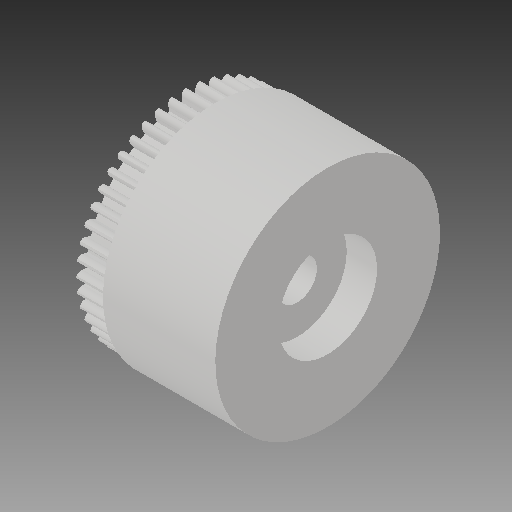
# Autodesk Inventor part: correct_wheel
Saved by Autodesk Inventor 2018 (Build 220112000, 112)
## iProperties
Created: 2017-11-06
Part Number: correct_wheel
Material: Generic
Document SubType Name: Modeling
Designer: kcmat
Density: 1 g/cm^3
Appearance: Default
Author: kcmat
Autodesk Inventor part; units mm, degrees
ref_plane "YZ Plane" through (0, 0, 0) normal (1, 0, 0) x (0, 1, 0)
ref_plane "XZ Plane" through (0, 0, 0) normal (0, 1, 0) x (-1, 0, 0)
ref_plane "XY Plane" through (0, 0, 0) normal (0, 0, 1) x (1, 0, 0)
sketch "Sketch1" plane through (0, 0, 0) normal (1, 0, 0) x (0, 1, 0)
  circle A0 centre (0, 0) radius 25.4
  circle A1 centre (0, 0) radius 4.445
  dimension "d3" = 8.89
  constraints: 2 centre point, 1 coincident
  measures "d3" diameter of A1
extrude "Extrusion1" add sketch "Sketch1" along normal blind 25.4
sketch "Sketch2" plane through (0, 0, 0) normal (-1, 0, 0) x (0, 0, 1)
  circle A0 centre (0, 0) radius 10.9855
  dimension "d6" = 21.971
  constraints: 1 centre point, 1 coincident
  measures "d6" diameter of A0
extrude "Extrusion2" cut sketch "Sketch2" against normal blind 6.858
sketch "Sketch3" plane through (25.4, 0, 0) normal (1, 0, 0) x (0, 0, -1)
  circle A0 centre (0, 0) radius 10.9855
  dimension "d9" = 21.971
  constraints: 1 centre point, 1 coincident
  measures "d9" diameter of A0
extrude "Extrusion3" cut sketch "Sketch3" against normal blind 6.858
sketch "Sketch4" plane through (0, 0, 0) normal (-1, 0, 0) x (0, 0, 1)
  circle A0 centre (0, 0) radius 10.9855
  circle A1 centre (0, 0) radius 10.9855 projected
  line L0 (-22.3513, -1.1327) -> (-22.3431, -1.1327) construction
  arc A2 (-24.7744, 0.2429) -> (-24.7744, -0.246) centre (-0.1732, -0.0016) ccw
  line L1 (-22.38, 1.002) -> (-22.3575, 0.9992)
  circle A3 centre (-0.1732, -0.0016) radius 22.2128
  arc A4 (-22.38, 0.5127) -> (-22.38, -0.5158) centre (-0.1732, -0.0016) ccw
  arc A5 (-24.7744, -0.246) -> (-23.3358, -0.7286) centre (-23.7217, 0.5066) ccw
  line L2 (-23.3358, -0.7286) -> (-22.3763, -0.6565)
  arc A6 (-23.3358, 0.7254) -> (-24.7744, 0.2429) centre (-23.7217, -0.5097) ccw
  line L3 (-23.3358, 0.7254) -> (-22.3763, 0.6534)
  arc A7 (-22.3763, 0.6534) -> (-22.3763, -0.6565) centre (-0.1732, -0.0016) ccw
  line L4 (-22.0139, -4.0179) -> (-22.0057, -4.0168) construction
  arc A8 (-22.2571, -2.3903) -> (-22.1229, -3.41) centre (-0.1732, -0.0016) ccw
  arc A9 (-22.2718, -2.2503) -> (-22.1009, -3.549) centre (-0.1732, -0.0016) ccw
  line L5 (-23.0427, -3.7457) -> (-22.1009, -3.549)
  line L6 (-23.2325, -2.3041) -> (-22.2718, -2.2503)
  arc A10 (-24.5321, -3.4551) -> (-23.0427, -3.7457) centre (-23.5866, -2.5715) ccw
  arc A11 (-24.5959, -2.9703) -> (-24.5321, -3.4551) centre (-0.1732, -0.0016) ccw
  arc A12 (-23.2325, -2.3041) -> (-24.5959, -2.9703) centre (-23.454, -3.5791) ccw
  line L7 (-22.321, -1.9052) -> (-22.2984, -1.905)
  line L8 (-21.3028, -6.8343) -> (-21.2949, -6.8322) construction
  arc A13 (-21.7564, -5.2524) -> (-21.4902, -6.2458) centre (-0.1732, -0.0016) ccw
  arc A14 (-21.7892, -5.1156) -> (-21.4502, -6.3807) centre (-0.1732, -0.0016) ccw
  line L9 (-22.3583, -6.6987) -> (-21.4502, -6.3807)
  line L10 (-22.7347, -5.2942) -> (-21.7892, -5.1156)
  arc A15 (-23.8729, -6.605) -> (-22.3583, -6.6987) centre (-23.0509, -5.6055) ccw
  arc A16 (-23.9994, -6.1327) -> (-23.8729, -6.605) centre (-0.1732, -0.0016) ccw
  arc A17 (-22.7347, -5.2942) -> (-23.9994, -6.1327) centre (-22.7878, -6.5872) ccw
  line L11 (-21.8831, -4.7797) -> (-21.8607, -4.7766)
  line L12 (-20.2302, -9.5338) -> (-20.2226, -9.5307) construction
  arc A18 (-20.8864, -8.0247) -> (-20.4928, -8.9748) centre (-0.1732, -0.0016) ccw
  arc A19 (-20.9368, -7.8933) -> (-20.4356, -9.1034) centre (-0.1732, -0.0016) ccw
  line L13 (-21.2944, -9.5372) -> (-20.4356, -9.1034)
  line L14 (-21.8508, -8.1938) -> (-20.9368, -7.8933)
  arc A20 (-22.8082, -9.6419) -> (-21.2944, -9.5372) centre (-22.1237, -8.5437) ccw
  arc A21 (-22.9953, -9.1902) -> (-22.8082, -9.6419) centre (-0.1732, -0.0016) ccw
  arc A22 (-21.8508, -8.1938) -> (-22.9953, -9.1902) centre (-21.7348, -9.4827) ccw
  line L15 (-21.0737, -7.5726) -> (-21.0518, -7.5665)
  line L16 (-18.8144, -12.0703) -> (-18.8073, -12.0661) construction
  arc A23 (-19.662, -10.6596) -> (-19.1477, -11.5503) centre (-0.1732, -0.0016) ccw
  arc A24 (-19.7291, -10.5359) -> (-19.0742, -11.6703) centre (-0.1732, -0.0016) ccw
  line L17 (-19.8691, -12.2125) -> (-19.0742, -11.6703)
  line L18 (-20.5961, -10.9532) -> (-19.7291, -10.5359)
  arc A25 (-21.3562, -12.5139) -> (-19.8691, -12.2125) centre (-20.8209, -11.3358) ccw
  arc A26 (-21.6007, -12.0905) -> (-21.3562, -12.5139) centre (-0.1732, -0.0016) ccw
  arc A27 (-20.5961, -10.9532) -> (-21.6007, -12.0905) centre (-20.3128, -12.2159) ccw
  line L19 (-19.9066, -10.2359) -> (-19.8858, -10.227)
  line L20 (-17.0796, -14.4002) -> (-17.0731, -14.3952) construction
  arc A28 (-18.1041, -13.1123) -> (-17.478, -13.9282) centre (-0.1732, -0.0016) ccw
  arc A29 (-18.1868, -12.9984) -> (-17.3894, -14.0375) centre (-0.1732, -0.0016) ccw
  line L21 (-18.1067, -14.6788) -> (-17.3894, -14.0375)
  line L22 (-18.9919, -13.5253) -> (-18.1868, -12.9984)
  arc A30 (-19.5418, -15.1718) -> (-18.1067, -14.6788) centre (-19.1649, -13.9339) ccw
  arc A31 (-19.8395, -14.7839) -> (-19.5418, -15.1718) centre (-0.1732, -0.0016) ccw
  arc A32 (-18.9919, -13.5253) -> (-19.8395, -14.7839) centre (-18.5462, -14.7402) ccw
  line L23 (-18.402, -12.724) -> (-18.3825, -12.7126)
  line L24 (-15.0556, -16.4837) -> (-15.0498, -16.4779) construction
  arc A33 (-16.2394, -15.3405) -> (-15.5122, -16.0678) centre (-0.1732, -0.0016) ccw
  arc A34 (-16.3362, -15.2384) -> (-15.4101, -16.1646) centre (-0.1732, -0.0016) ccw
  line L25 (-16.0375, -16.894) -> (-15.4101, -16.1646)
  line L26 (-17.0657, -15.8659) -> (-16.3362, -15.2384)
  arc A35 (-17.396, -17.5701) -> (-16.0375, -16.894) centre (-17.1838, -16.2936) ccw
  arc A36 (-17.7418, -17.2244) -> (-17.396, -17.5701) centre (-0.1732, -0.0016) ccw
  arc A37 (-17.0657, -15.8659) -> (-17.7418, -17.2244) centre (-16.4652, -17.0122) ccw
  line L27 (-16.5854, -14.9945) -> (-16.5676, -14.9806)
  line L28 (-12.7769, -18.2853) -> (-12.7719, -18.2787) construction
  arc A38 (-14.0998, -17.3064) -> (-13.2839, -17.9325) centre (-0.1732, -0.0016) ccw
  arc A39 (-14.2092, -17.2178) -> (-13.17, -18.0152) centre (-0.1732, -0.0016) ccw
  line L29 (-13.6969, -18.8202) -> (-13.17, -18.0152)
  line L30 (-14.8504, -17.9351) -> (-14.2092, -17.2178)
  arc A40 (-14.9555, -19.6679) -> (-13.6969, -18.8202) centre (-14.9118, -18.3745) ccw
  arc A41 (-15.3434, -19.3702) -> (-14.9555, -19.6679) centre (-0.1732, -0.0016) ccw
  arc A42 (-14.8504, -17.9351) -> (-15.3434, -19.3702) centre (-14.1055, -18.9932) ccw
  line L31 (-14.488, -17.0085) -> (-14.4722, -16.9923)
  line L32 (-10.2826, -19.774) -> (-10.2785, -19.7668) construction
  arc A43 (-11.7219, -18.9761) -> (-10.8313, -19.4903) centre (-0.1732, -0.0016) ccw
  arc A44 (-11.8419, -18.9026) -> (-10.7076, -19.5575) centre (-0.1732, -0.0016) ccw
  line L33 (-11.1249, -20.4244) -> (-10.7076, -19.5575)
  line L34 (-12.3841, -19.6974) -> (-11.8419, -18.9026)
  arc A45 (-12.2621, -21.4291) -> (-11.1249, -20.4244) centre (-12.3875, -20.1411) ccw
  arc A46 (-12.6855, -21.1846) -> (-12.2621, -21.4291) centre (-0.1732, -0.0016) ccw
  arc A47 (-12.3841, -19.6974) -> (-12.6855, -21.1846) centre (-11.5074, -20.6493) ccw
  line L35 (-12.1457, -18.7315) -> (-12.1321, -18.7134)
  line L36 (-7.6153, -20.9244) -> (-7.6121, -20.9167) construction
  arc A48 (-9.1464, -20.3212) -> (-8.1963, -20.7148) centre (-0.1732, -0.0016) ccw
  arc A49 (-9.275, -20.2639) -> (-8.0649, -20.7652) centre (-0.1732, -0.0016) ccw
  line L37 (-8.3654, -21.6792) -> (-8.0649, -20.7652)
  line L38 (-9.7088, -21.1228) -> (-9.275, -20.2639)
  arc A50 (-9.3618, -22.8237) -> (-8.3654, -21.6792) centre (-9.6543, -21.5631) ccw
  arc A51 (-9.8135, -22.6366) -> (-9.3618, -22.8237) centre (-0.1732, -0.0016) ccw
  arc A52 (-9.7088, -21.1228) -> (-9.8135, -22.6366) centre (-8.7153, -21.9521) ccw
  line L39 (-9.5985, -20.1339) -> (-9.5874, -20.1142)
  line L40 (-4.8207, -21.7168) -> (-4.8185, -21.7088) construction
  arc A53 (-6.4174, -21.3186) -> (-5.424, -21.5848) centre (-0.1732, -0.0016) ccw
  arc A54 (-6.5524, -21.2786) -> (-5.2872, -21.6176) centre (-0.1732, -0.0016) ccw
  line L41 (-5.4659, -22.5631) -> (-5.2872, -21.6176)
  line L42 (-6.8703, -22.1867) -> (-6.5524, -21.2786)
  arc A55 (-6.3043, -23.8278) -> (-5.4659, -22.5631) centre (-6.7588, -22.6162) ccw
  arc A56 (-6.7766, -23.7013) -> (-6.3043, -23.8278) centre (-0.1732, -0.0016) ccw
  arc A57 (-6.8703, -22.1867) -> (-6.7766, -23.7013) centre (-5.7772, -22.8792) ccw
  line L43 (-6.8901, -21.192) -> (-6.8816, -21.171)
  line L44 (-1.9465, -22.1376) -> (-1.9454, -22.1294) construction
  arc A58 (-3.5816, -21.9513) -> (-2.5619, -22.0855) centre (-0.1732, -0.0016) ccw
  arc A59 (-3.7206, -21.9292) -> (-2.422, -22.1002) centre (-0.1732, -0.0016) ccw
  line L45 (-2.4757, -23.0609) -> (-2.422, -22.1002)
  line L46 (-3.9173, -22.8711) -> (-3.7206, -21.9292)
  arc A60 (-3.1419, -24.4243) -> (-2.4757, -23.0609) centre (-3.7507, -23.2823) ccw
  arc A61 (-3.6267, -24.3604) -> (-3.1419, -24.4243) centre (-0.1732, -0.0016) ccw
  arc A62 (-3.9173, -22.8711) -> (-3.6267, -24.3604) centre (-2.7431, -23.415) ccw
  line L47 (-4.0667, -21.8874) -> (-4.0611, -21.8655)
  line L48 (0.958, -22.1797) -> (0.958, -22.1714) construction
  arc A63 (-0.6874, -22.2084) -> (0.341, -22.2084) centre (-0.1732, -0.0016) ccw
  arc A64 (-0.8281, -22.2047) -> (0.4817, -22.2047) centre (-0.1732, -0.0016) ccw
  line L49 (0.5538, -23.1641) -> (0.4817, -22.2047)
  line L50 (-0.9002, -23.1641) -> (-0.8281, -22.2047)
  arc A65 (0.0713, -24.6028) -> (0.5538, -23.1641) centre (-0.6813, -23.5501) ccw
  arc A66 (-0.4177, -24.6028) -> (0.0713, -24.6028) centre (-0.1732, -0.0016) ccw
  arc A67 (-0.9002, -23.1641) -> (-0.4177, -24.6028) centre (0.335, -23.5501) ccw
  line L51 (-1.1767, -22.2084) -> (-1.174, -22.1859)
  line L52 (3.8432, -21.8423) -> (3.8421, -21.8341) construction
  arc A68 (2.2156, -22.0855) -> (3.2352, -21.9513) centre (-0.1732, -0.0016) ccw
  arc A69 (2.0756, -22.1002) -> (3.3742, -21.9292) centre (-0.1732, -0.0016) ccw
  line L53 (3.5709, -22.8711) -> (3.3742, -21.9292)
  line L54 (2.1294, -23.0609) -> (2.0756, -22.1002)
  arc A70 (3.2803, -24.3604) -> (3.5709, -22.8711) centre (2.3967, -23.415) ccw
  arc A71 (2.7955, -24.4243) -> (3.2803, -24.3604) centre (-0.1732, -0.0016) ccw
  arc A72 (2.1294, -23.0609) -> (2.7955, -24.4243) centre (3.4043, -23.2823) ccw
  line L55 (1.7304, -22.1494) -> (1.7302, -22.1268)
  line L56 (6.6596, -21.1312) -> (6.6575, -21.1232) construction
  arc A73 (5.0777, -21.5848) -> (6.0711, -21.3186) centre (-0.1732, -0.0016) ccw
  arc A74 (4.9408, -21.6176) -> (6.206, -21.2786) centre (-0.1732, -0.0016) ccw
  line L57 (6.524, -22.1867) -> (6.206, -21.2786)
  line L58 (5.1195, -22.5631) -> (4.9408, -21.6176)
  arc A75 (6.4302, -23.7013) -> (6.524, -22.1867) centre (5.4308, -22.8792) ccw
  arc A76 (5.9579, -23.8278) -> (6.4302, -23.7013) centre (-0.1732, -0.0016) ccw
  arc A77 (5.1195, -22.5631) -> (5.9579, -23.8278) centre (6.4125, -22.6162) ccw
  line L59 (4.605, -21.7114) -> (4.6019, -21.689)
  line L60 (9.3591, -20.0586) -> (9.356, -20.051) construction
  arc A78 (7.8499, -20.7148) -> (8.8001, -20.3212) centre (-0.1732, -0.0016) ccw
  arc A79 (7.7185, -20.7652) -> (8.9286, -20.2639) centre (-0.1732, -0.0016) ccw
  line L61 (9.3624, -21.1228) -> (8.9286, -20.2639)
  line L62 (8.0191, -21.6792) -> (7.7185, -20.7652)
  arc A80 (9.4672, -22.6366) -> (9.3624, -21.1228) centre (8.369, -21.9521) ccw
  arc A81 (9.0154, -22.8237) -> (9.4672, -22.6366) centre (-0.1732, -0.0016) ccw
  arc A82 (8.0191, -21.6792) -> (9.0154, -22.8237) centre (9.3079, -21.5631) ccw
  line L63 (7.3978, -20.902) -> (7.3918, -20.8802)
  line L64 (11.8955, -18.6428) -> (11.8914, -18.6356) construction
  arc A83 (10.4849, -19.4903) -> (11.3756, -18.9761) centre (-0.1732, -0.0016) ccw
  arc A84 (10.3612, -19.5575) -> (11.4956, -18.9026) centre (-0.1732, -0.0016) ccw
  line L65 (12.0377, -19.6974) -> (11.4956, -18.9026)
  line L66 (10.7785, -20.4244) -> (10.3612, -19.5575)
  arc A85 (12.3392, -21.1846) -> (12.0377, -19.6974) centre (11.161, -20.6493) ccw
  arc A86 (11.9157, -21.4291) -> (12.3392, -21.1846) centre (-0.1732, -0.0016) ccw
  arc A87 (10.7785, -20.4244) -> (11.9157, -21.4291) centre (12.0412, -20.1411) ccw
  line L67 (10.0611, -19.735) -> (10.0523, -19.7142)
  line L68 (14.2254, -16.908) -> (14.2204, -16.9015) construction
  arc A88 (12.9375, -17.9325) -> (13.7534, -17.3064) centre (-0.1732, -0.0016) ccw
  arc A89 (12.8236, -18.0152) -> (13.8628, -17.2178) centre (-0.1732, -0.0016) ccw
  line L69 (14.5041, -17.9351) -> (13.8628, -17.2178)
  line L70 (13.3505, -18.8202) -> (12.8236, -18.0152)
  arc A90 (14.9971, -19.3702) -> (14.5041, -17.9351) centre (13.7591, -18.9932) ccw
  arc A91 (14.6092, -19.6679) -> (14.9971, -19.3702) centre (-0.1732, -0.0016) ccw
  arc A92 (13.3505, -18.8202) -> (14.6092, -19.6679) centre (14.5654, -18.3745) ccw
  line L71 (12.5493, -18.2303) -> (12.5378, -18.2108)
  line L72 (16.309, -14.884) -> (16.3032, -14.8782) construction
  arc A93 (15.1658, -16.0678) -> (15.893, -15.3405) centre (-0.1732, -0.0016) ccw
  arc A94 (15.0637, -16.1646) -> (15.9899, -15.2384) centre (-0.1732, -0.0016) ccw
  line L73 (16.7193, -15.8659) -> (15.9899, -15.2384)
  line L74 (15.6912, -16.894) -> (15.0637, -16.1646)
  arc A95 (17.3954, -17.2244) -> (16.7193, -15.8659) centre (16.1189, -17.0122) ccw
  arc A96 (17.0497, -17.5701) -> (17.3954, -17.2244) centre (-0.1732, -0.0016) ccw
  arc A97 (15.6912, -16.894) -> (17.0497, -17.5701) centre (16.8375, -16.2936) ccw
  line L75 (14.8198, -16.4138) -> (14.8059, -16.3959)
  line L76 (18.1105, -12.6053) -> (18.104, -12.6003) construction
  arc A98 (17.1316, -13.9282) -> (17.7577, -13.1123) centre (-0.1732, -0.0016) ccw
  arc A99 (17.0431, -14.0375) -> (17.8404, -12.9984) centre (-0.1732, -0.0016) ccw
  line L77 (18.6455, -13.5253) -> (17.8404, -12.9984)
  line L78 (17.7604, -14.6788) -> (17.0431, -14.0375)
  arc A100 (19.4931, -14.7839) -> (18.6455, -13.5253) centre (18.1998, -14.7402) ccw
  arc A101 (19.1955, -15.1718) -> (19.4931, -14.7839) centre (-0.1732, -0.0016) ccw
  arc A102 (17.7604, -14.6788) -> (19.1955, -15.1718) centre (18.8185, -13.9339) ccw
  line L79 (16.8338, -14.3164) -> (16.8176, -14.3005)
  line L80 (19.5992, -10.111) -> (19.5921, -10.1069) construction
  arc A103 (18.8014, -11.5503) -> (19.3156, -10.6596) centre (-0.1732, -0.0016) ccw
  arc A104 (18.7278, -11.6703) -> (19.3827, -10.5359) centre (-0.1732, -0.0016) ccw
  line L81 (20.2497, -10.9532) -> (19.3827, -10.5359)
  line L82 (19.5227, -12.2125) -> (18.7278, -11.6703)
  arc A105 (21.2544, -12.0905) -> (20.2497, -10.9532) centre (19.9664, -12.2159) ccw
  arc A106 (21.0099, -12.5139) -> (21.2544, -12.0905) centre (-0.1732, -0.0016) ccw
  arc A107 (19.5227, -12.2125) -> (21.0099, -12.5139) centre (20.4746, -11.3358) ccw
  line L83 (18.5567, -11.9741) -> (18.5386, -11.9605)
  line L84 (20.7496, -7.4437) -> (20.742, -7.4405) construction
  arc A108 (20.1465, -8.9748) -> (20.54, -8.0247) centre (-0.1732, -0.0016) ccw
  arc A109 (20.0892, -9.1034) -> (20.5905, -7.8933) centre (-0.1732, -0.0016) ccw
  line L85 (21.5045, -8.1938) -> (20.5905, -7.8933)
  line L86 (20.948, -9.5372) -> (20.0892, -9.1034)
  arc A110 (22.649, -9.1902) -> (21.5045, -8.1938) centre (21.3884, -9.4827) ccw
  arc A111 (22.4619, -9.6419) -> (22.649, -9.1902) centre (-0.1732, -0.0016) ccw
  arc A112 (20.948, -9.5372) -> (22.4619, -9.6419) centre (21.7773, -8.5437) ccw
  line L87 (19.9592, -9.4269) -> (19.9395, -9.4158)
  line L88 (21.542, -4.649) -> (21.5341, -4.6469) construction
  arc A113 (21.1439, -6.2458) -> (21.4101, -5.2524) centre (-0.1732, -0.0016) ccw
  arc A114 (21.1039, -6.3807) -> (21.4429, -5.1156) centre (-0.1732, -0.0016) ccw
  line L89 (22.3883, -5.2942) -> (21.4429, -5.1156)
  line L90 (22.012, -6.6987) -> (21.1039, -6.3807)
  arc A115 (23.6531, -6.1327) -> (22.3883, -5.2942) centre (22.4415, -6.5872) ccw
  arc A116 (23.5265, -6.605) -> (23.6531, -6.1327) centre (-0.1732, -0.0016) ccw
  arc A117 (22.012, -6.6987) -> (23.5265, -6.605) centre (22.7045, -5.6055) ccw
  line L91 (21.0172, -6.7185) -> (20.9962, -6.71)
  line L92 (21.9629, -1.7749) -> (21.9547, -1.7738) construction
  arc A118 (21.7765, -3.41) -> (21.9108, -2.3903) centre (-0.1732, -0.0016) ccw
  arc A119 (21.7545, -3.549) -> (21.9255, -2.2503) centre (-0.1732, -0.0016) ccw
  line L93 (22.8861, -2.3041) -> (21.9255, -2.2503)
  line L94 (22.6964, -3.7457) -> (21.7545, -3.549)
  arc A120 (24.2495, -2.9703) -> (22.8861, -2.3041) centre (23.1076, -3.5791) ccw
  arc A121 (24.1857, -3.4551) -> (24.2495, -2.9703) centre (-0.1732, -0.0016) ccw
  arc A122 (22.6964, -3.7457) -> (24.1857, -3.4551) centre (23.2403, -2.5715) ccw
  line L95 (21.7127, -3.8951) -> (21.6908, -3.8894)
  line L96 (22.005, 1.1296) -> (21.9967, 1.1296) construction
  arc A123 (22.0336, -0.5158) -> (22.0336, 0.5127) centre (-0.1732, -0.0016) ccw
  arc A124 (22.0299, -0.6565) -> (22.0299, 0.6534) centre (-0.1732, -0.0016) ccw
  line L97 (22.9894, 0.7254) -> (22.0299, 0.6534)
  line L98 (22.9894, -0.7286) -> (22.0299, -0.6565)
  arc A125 (24.4281, 0.2429) -> (22.9894, 0.7254) centre (23.3754, -0.5097) ccw
  arc A126 (24.4281, -0.246) -> (24.4281, 0.2429) centre (-0.1732, -0.0016) ccw
  arc A127 (22.9894, -0.7286) -> (24.4281, -0.246) centre (23.3754, 0.5066) ccw
  line L99 (22.0336, -1.0051) -> (22.0112, -1.0024)
  line L100 (21.6676, 4.0148) -> (21.6594, 4.0137) construction
  arc A128 (21.9108, 2.3872) -> (21.7765, 3.4068) centre (-0.1732, -0.0016) ccw
  arc A129 (21.9255, 2.2472) -> (21.7545, 3.5458) centre (-0.1732, -0.0016) ccw
  line L101 (22.6964, 3.7426) -> (21.7545, 3.5458)
  line L102 (22.8861, 2.301) -> (21.9255, 2.2472)
  arc A130 (24.1857, 3.4519) -> (22.6964, 3.7426) centre (23.2403, 2.5683) ccw
  arc A131 (24.2495, 2.9672) -> (24.1857, 3.4519) centre (-0.1732, -0.0016) ccw
  arc A132 (22.8861, 2.301) -> (24.2495, 2.9672) centre (23.1076, 3.576) ccw
  line L103 (21.9747, 1.902) -> (21.952, 1.9018)
  line L104 (20.9565, 6.8312) -> (20.9485, 6.8291) construction
  arc A133 (21.4101, 5.2493) -> (21.1439, 6.2427) centre (-0.1732, -0.0016) ccw
  arc A134 (21.4429, 5.1124) -> (21.1039, 6.3776) centre (-0.1732, -0.0016) ccw
  line L105 (22.012, 6.6956) -> (21.1039, 6.3776)
  line L106 (22.3883, 5.2911) -> (21.4429, 5.1124)
  arc A135 (23.5265, 6.6019) -> (22.012, 6.6956) centre (22.7045, 5.6024) ccw
  arc A136 (23.6531, 6.1296) -> (23.5265, 6.6019) centre (-0.1732, -0.0016) ccw
  arc A137 (22.3883, 5.2911) -> (23.6531, 6.1296) centre (22.4415, 6.5841) ccw
  line L107 (21.5367, 4.7766) -> (21.5143, 4.7735)
  line L108 (19.8839, 9.5307) -> (19.8762, 9.5276) construction
  arc A138 (20.54, 8.0215) -> (20.1465, 8.9717) centre (-0.1732, -0.0016) ccw
  arc A139 (20.5905, 7.8901) -> (20.0892, 9.1003) centre (-0.1732, -0.0016) ccw
  line L109 (20.948, 9.534) -> (20.0892, 9.1003)
  line L110 (21.5045, 8.1907) -> (20.5905, 7.8901)
  arc A140 (22.4619, 9.6388) -> (20.948, 9.534) centre (21.7773, 8.5406) ccw
  arc A141 (22.649, 9.1871) -> (22.4619, 9.6388) centre (-0.1732, -0.0016) ccw
  arc A142 (21.5045, 8.1907) -> (22.649, 9.1871) centre (21.3884, 9.4796) ccw
  line L111 (20.7273, 7.5695) -> (20.7055, 7.5634)
  line L112 (18.4681, 12.0671) -> (18.4609, 12.063) construction
  arc A143 (19.3156, 10.6565) -> (18.8014, 11.5472) centre (-0.1732, -0.0016) ccw
  arc A144 (19.3827, 10.5328) -> (18.7278, 11.6672) centre (-0.1732, -0.0016) ccw
  line L113 (19.5227, 12.2093) -> (18.7278, 11.6672)
  line L114 (20.2497, 10.9501) -> (19.3827, 10.5328)
  arc A145 (21.0099, 12.5108) -> (19.5227, 12.2093) centre (20.4746, 11.3326) ccw
  arc A146 (21.2544, 12.0873) -> (21.0099, 12.5108) centre (-0.1732, -0.0016) ccw
  arc A147 (20.2497, 10.9501) -> (21.2544, 12.0873) centre (19.9664, 12.2128) ccw
  line L115 (19.5603, 10.2327) -> (19.5394, 10.2239)
  line L116 (16.7333, 14.3971) -> (16.7268, 14.392) construction
  arc A148 (17.7577, 13.1091) -> (17.1316, 13.9251) centre (-0.1732, -0.0016) ccw
  arc A149 (17.8404, 12.9953) -> (17.0431, 14.0344) centre (-0.1732, -0.0016) ccw
  line L117 (17.7604, 14.6757) -> (17.0431, 14.0344)
  line L118 (18.6455, 13.5222) -> (17.8404, 12.9953)
  arc A150 (19.1955, 15.1687) -> (17.7604, 14.6757) centre (18.8185, 13.9308) ccw
  arc A151 (19.4931, 14.7808) -> (19.1955, 15.1687) centre (-0.1732, -0.0016) ccw
  arc A152 (18.6455, 13.5222) -> (19.4931, 14.7808) centre (18.1998, 14.737) ccw
  line L119 (18.0556, 12.7209) -> (18.0361, 12.7094)
  line L120 (14.7093, 16.4806) -> (14.7034, 16.4748) construction
  arc A153 (15.893, 15.3374) -> (15.1658, 16.0646) centre (-0.1732, -0.0016) ccw
  arc A154 (15.9899, 15.2353) -> (15.0637, 16.1615) centre (-0.1732, -0.0016) ccw
  line L121 (15.6912, 16.8909) -> (15.0637, 16.1615)
  line L122 (16.7193, 15.8628) -> (15.9899, 15.2353)
  arc A155 (17.0497, 17.567) -> (15.6912, 16.8909) centre (16.8375, 16.2905) ccw
  arc A156 (17.3954, 17.2213) -> (17.0497, 17.567) centre (-0.1732, -0.0016) ccw
  arc A157 (16.7193, 15.8628) -> (17.3954, 17.2213) centre (16.1189, 17.0091) ccw
  line L123 (16.239, 14.9914) -> (16.2212, 14.9775)
  line L124 (12.4306, 18.2822) -> (12.4256, 18.2756) construction
  arc A158 (13.7534, 17.3033) -> (12.9375, 17.9293) centre (-0.1732, -0.0016) ccw
  arc A159 (13.8628, 17.2147) -> (12.8236, 18.012) centre (-0.1732, -0.0016) ccw
  line L125 (13.3505, 18.8171) -> (12.8236, 18.012)
  line L126 (14.5041, 17.932) -> (13.8628, 17.2147)
  arc A160 (14.6092, 19.6648) -> (13.3505, 18.8171) centre (14.5654, 18.3714) ccw
  arc A161 (14.9971, 19.3671) -> (14.6092, 19.6648) centre (-0.1732, -0.0016) ccw
  arc A162 (14.5041, 17.932) -> (14.9971, 19.3671) centre (13.7591, 18.9901) ccw
  line L127 (14.1417, 17.0054) -> (14.1258, 16.9892)
  line L128 (9.9362, 19.7709) -> (9.9321, 19.7637) construction
  arc A163 (11.3756, 18.973) -> (10.4849, 19.4872) centre (-0.1732, -0.0016) ccw
  arc A164 (11.4956, 18.8995) -> (10.3612, 19.5544) centre (-0.1732, -0.0016) ccw
  line L129 (10.7785, 20.4213) -> (10.3612, 19.5544)
  line L130 (12.0377, 19.6943) -> (11.4956, 18.8995)
  arc A165 (11.9157, 21.426) -> (10.7785, 20.4213) centre (12.0412, 20.138) ccw
  arc A166 (12.3392, 21.1815) -> (11.9157, 21.426) centre (-0.1732, -0.0016) ccw
  arc A167 (12.0377, 19.6943) -> (12.3392, 21.1815) centre (11.161, 20.6462) ccw
  line L131 (11.7993, 18.7283) -> (11.7857, 18.7103)
  line L132 (7.2689, 20.9212) -> (7.2658, 20.9136) construction
  arc A168 (8.8001, 20.3181) -> (7.8499, 20.7117) centre (-0.1732, -0.0016) ccw
  arc A169 (8.9286, 20.2608) -> (7.7185, 20.7621) centre (-0.1732, -0.0016) ccw
  line L133 (8.0191, 21.6761) -> (7.7185, 20.7621)
  line L134 (9.3624, 21.1197) -> (8.9286, 20.2608)
  arc A170 (9.0154, 22.8206) -> (8.0191, 21.6761) centre (9.3079, 21.56) ccw
  arc A171 (9.4672, 22.6335) -> (9.0154, 22.8206) centre (-0.1732, -0.0016) ccw
  arc A172 (9.3624, 21.1197) -> (9.4672, 22.6335) centre (8.369, 21.9489) ccw
  line L135 (9.2522, 20.1308) -> (9.241, 20.1111)
  line L136 (4.4743, 21.7136) -> (4.4722, 21.7057) construction
  arc A173 (6.0711, 21.3155) -> (5.0777, 21.5817) centre (-0.1732, -0.0016) ccw
  arc A174 (6.206, 21.2755) -> (4.9408, 21.6145) centre (-0.1732, -0.0016) ccw
  line L137 (5.1195, 22.5599) -> (4.9408, 21.6145)
  line L138 (6.524, 22.1836) -> (6.206, 21.2755)
  arc A175 (5.9579, 23.8247) -> (5.1195, 22.5599) centre (6.4125, 22.6131) ccw
  arc A176 (6.4302, 23.6981) -> (5.9579, 23.8247) centre (-0.1732, -0.0016) ccw
  arc A177 (6.524, 22.1836) -> (6.4302, 23.6981) centre (5.4308, 22.8761) ccw
  line L139 (6.5437, 21.1888) -> (6.5353, 21.1679)
  line L140 (1.6001, 22.1345) -> (1.5991, 22.1263) construction
  arc A178 (3.2352, 21.9482) -> (2.2156, 22.0824) centre (-0.1732, -0.0016) ccw
  arc A179 (3.3742, 21.9261) -> (2.0756, 22.0971) centre (-0.1732, -0.0016) ccw
  line L141 (2.1294, 23.0578) -> (2.0756, 22.0971)
  line L142 (3.5709, 22.868) -> (3.3742, 21.9261)
  arc A180 (2.7955, 24.4211) -> (2.1294, 23.0578) centre (3.4043, 23.2792) ccw
  arc A181 (3.2803, 24.3573) -> (2.7955, 24.4211) centre (-0.1732, -0.0016) ccw
  arc A182 (3.5709, 22.868) -> (3.2803, 24.3573) centre (2.3967, 23.4119) ccw
  line L143 (3.7204, 21.8843) -> (3.7147, 21.8624)
  line L144 (-1.3044, 22.1766) -> (-1.3044, 22.1683) construction
  arc A183 (0.341, 22.2053) -> (-0.6874, 22.2053) centre (-0.1732, -0.0016) ccw
  arc A184 (0.4817, 22.2016) -> (-0.8281, 22.2016) centre (-0.1732, -0.0016) ccw
  line L145 (-0.9002, 23.161) -> (-0.8281, 22.2016)
  line L146 (0.5538, 23.161) -> (0.4817, 22.2016)
  arc A185 (-0.4177, 24.5997) -> (-0.9002, 23.161) centre (0.335, 23.547) ccw
  arc A186 (0.0713, 24.5997) -> (-0.4177, 24.5997) centre (-0.1732, -0.0016) ccw
  arc A187 (0.5538, 23.161) -> (0.0713, 24.5997) centre (-0.6813, 23.547) ccw
  line L147 (0.8304, 22.2053) -> (0.8276, 22.1828)
  line L148 (-4.1895, 21.8392) -> (-4.1884, 21.831) construction
  arc A188 (-2.5619, 22.0824) -> (-3.5816, 21.9482) centre (-0.1732, -0.0016) ccw
  arc A189 (-2.422, 22.0971) -> (-3.7206, 21.9261) centre (-0.1732, -0.0016) ccw
  line L149 (-3.9173, 22.868) -> (-3.7206, 21.9261)
  line L150 (-2.4757, 23.0578) -> (-2.422, 22.0971)
  arc A190 (-3.6267, 24.3573) -> (-3.9173, 22.868) centre (-2.7431, 23.4119) ccw
  arc A191 (-3.1419, 24.4211) -> (-3.6267, 24.3573) centre (-0.1732, -0.0016) ccw
  arc A192 (-2.4757, 23.0578) -> (-3.1419, 24.4211) centre (-3.7507, 23.2792) ccw
  line L151 (-2.0768, 22.1463) -> (-2.0766, 22.1236)
  line L152 (-7.0059, 21.1281) -> (-7.0038, 21.1201) construction
  arc A193 (-5.424, 21.5817) -> (-6.4174, 21.3155) centre (-0.1732, -0.0016) ccw
  arc A194 (-5.2872, 21.6145) -> (-6.5524, 21.2755) centre (-0.1732, -0.0016) ccw
  line L153 (-6.8703, 22.1836) -> (-6.5524, 21.2755)
  line L154 (-5.4659, 22.5599) -> (-5.2872, 21.6145)
  arc A195 (-6.7766, 23.6981) -> (-6.8703, 22.1836) centre (-5.7772, 22.8761) ccw
  arc A196 (-6.3043, 23.8247) -> (-6.7766, 23.6981) centre (-0.1732, -0.0016) ccw
  arc A197 (-5.4659, 22.5599) -> (-6.3043, 23.8247) centre (-6.7588, 22.6131) ccw
  line L155 (-4.9514, 21.7083) -> (-4.9482, 21.6859)
  line L156 (-9.7055, 20.0555) -> (-9.7023, 20.0479) construction
  arc A198 (-8.1963, 20.7117) -> (-9.1464, 20.3181) centre (-0.1732, -0.0016) ccw
  arc A199 (-8.0649, 20.7621) -> (-9.275, 20.2608) centre (-0.1732, -0.0016) ccw
  line L157 (-9.7088, 21.1197) -> (-9.275, 20.2608)
  line L158 (-8.3654, 21.6761) -> (-8.0649, 20.7621)
  arc A200 (-9.8135, 22.6335) -> (-9.7088, 21.1197) centre (-8.7153, 21.9489) ccw
  arc A201 (-9.3618, 22.8206) -> (-9.8135, 22.6335) centre (-0.1732, -0.0016) ccw
  arc A202 (-8.3654, 21.6761) -> (-9.3618, 22.8206) centre (-9.6543, 21.56) ccw
  line L159 (-7.7442, 20.8989) -> (-7.7381, 20.8771)
  line L160 (-12.2419, 18.6397) -> (-12.2378, 18.6325) construction
  arc A203 (-10.8313, 19.4872) -> (-11.7219, 18.973) centre (-0.1732, -0.0016) ccw
  arc A204 (-10.7076, 19.5544) -> (-11.8419, 18.8995) centre (-0.1732, -0.0016) ccw
  line L161 (-12.3841, 19.6943) -> (-11.8419, 18.8995)
  line L162 (-11.1249, 20.4213) -> (-10.7076, 19.5544)
  arc A205 (-12.6855, 21.1815) -> (-12.3841, 19.6943) centre (-11.5074, 20.6462) ccw
  arc A206 (-12.2621, 21.426) -> (-12.6855, 21.1815) centre (-0.1732, -0.0016) ccw
  arc A207 (-11.1249, 20.4213) -> (-12.2621, 21.426) centre (-12.3875, 20.138) ccw
  line L163 (-10.4075, 19.7319) -> (-10.3986, 19.7111)
  line L164 (-14.5718, 16.9049) -> (-14.5668, 16.8984) construction
  arc A208 (-13.2839, 17.9293) -> (-14.0998, 17.3033) centre (-0.1732, -0.0016) ccw
  arc A209 (-13.17, 18.012) -> (-14.2092, 17.2147) centre (-0.1732, -0.0016) ccw
  line L165 (-14.8504, 17.932) -> (-14.2092, 17.2147)
  line L166 (-13.6969, 18.8171) -> (-13.17, 18.012)
  arc A210 (-15.3434, 19.3671) -> (-14.8504, 17.932) centre (-14.1055, 18.9901) ccw
  arc A211 (-14.9555, 19.6648) -> (-15.3434, 19.3671) centre (-0.1732, -0.0016) ccw
  arc A212 (-13.6969, 18.8171) -> (-14.9555, 19.6648) centre (-14.9118, 18.3714) ccw
  line L167 (-12.8957, 18.2272) -> (-12.8842, 18.2077)
  line L168 (-16.6554, 14.8809) -> (-16.6495, 14.875) construction
  arc A213 (-15.5122, 16.0646) -> (-16.2394, 15.3374) centre (-0.1732, -0.0016) ccw
  arc A214 (-15.4101, 16.1615) -> (-16.3362, 15.2353) centre (-0.1732, -0.0016) ccw
  line L169 (-17.0657, 15.8628) -> (-16.3362, 15.2353)
  line L170 (-16.0375, 16.8909) -> (-15.4101, 16.1615)
  arc A215 (-17.7418, 17.2213) -> (-17.0657, 15.8628) centre (-16.4652, 17.0091) ccw
  arc A216 (-17.396, 17.567) -> (-17.7418, 17.2213) centre (-0.1732, -0.0016) ccw
  arc A217 (-16.0375, 16.8909) -> (-17.396, 17.567) centre (-17.1838, 16.2905) ccw
  line L171 (-15.1661, 16.4107) -> (-15.1522, 16.3928)
  line L172 (-18.4569, 12.6022) -> (-18.4504, 12.5972) construction
  arc A218 (-17.478, 13.9251) -> (-18.1041, 13.1091) centre (-0.1732, -0.0016) ccw
  arc A219 (-17.3894, 14.0344) -> (-18.1868, 12.9953) centre (-0.1732, -0.0016) ccw
  line L173 (-18.9919, 13.5222) -> (-18.1868, 12.9953)
  line L174 (-18.1067, 14.6757) -> (-17.3894, 14.0344)
  arc A220 (-19.8395, 14.7808) -> (-18.9919, 13.5222) centre (-18.5462, 14.737) ccw
  arc A221 (-19.5418, 15.1687) -> (-19.8395, 14.7808) centre (-0.1732, -0.0016) ccw
  arc A222 (-18.1067, 14.6757) -> (-19.5418, 15.1687) centre (-19.1649, 13.9308) ccw
  line L175 (-17.1801, 14.3133) -> (-17.164, 14.2974)
  line L176 (-19.9456, 10.1079) -> (-19.9385, 10.1037) construction
  arc A223 (-19.1477, 11.5472) -> (-19.662, 10.6565) centre (-0.1732, -0.0016) ccw
  arc A224 (-19.0742, 11.6672) -> (-19.7291, 10.5328) centre (-0.1732, -0.0016) ccw
  line L177 (-20.5961, 10.9501) -> (-19.7291, 10.5328)
  line L178 (-19.8691, 12.2093) -> (-19.0742, 11.6672)
  arc A225 (-21.6007, 12.0873) -> (-20.5961, 10.9501) centre (-20.3128, 12.2128) ccw
  arc A226 (-21.3562, 12.5108) -> (-21.6007, 12.0873) centre (-0.1732, -0.0016) ccw
  arc A227 (-19.8691, 12.2093) -> (-21.3562, 12.5108) centre (-20.8209, 11.3326) ccw
  line L179 (-18.9031, 11.971) -> (-18.885, 11.9573)
  line L180 (-21.096, 7.4406) -> (-21.0884, 7.4374) construction
  arc A228 (-20.4928, 8.9717) -> (-20.8864, 8.0215) centre (-0.1732, -0.0016) ccw
  arc A229 (-20.4356, 9.1003) -> (-20.9368, 7.8901) centre (-0.1732, -0.0016) ccw
  line L181 (-21.8508, 8.1907) -> (-20.9368, 7.8901)
  line L182 (-21.2944, 9.534) -> (-20.4356, 9.1003)
  arc A230 (-22.9953, 9.1871) -> (-21.8508, 8.1907) centre (-21.7348, 9.4796) ccw
  arc A231 (-22.8082, 9.6388) -> (-22.9953, 9.1871) centre (-0.1732, -0.0016) ccw
  arc A232 (-21.2944, 9.534) -> (-22.8082, 9.6388) centre (-22.1237, 8.5406) ccw
  line L183 (-20.3056, 9.4238) -> (-20.2859, 9.4127)
  line L184 (-21.8884, 4.6459) -> (-21.8804, 4.6438) construction
  arc A233 (-21.4902, 6.2427) -> (-21.7564, 5.2493) centre (-0.1732, -0.0016) ccw
  arc A234 (-21.4502, 6.3776) -> (-21.7892, 5.1124) centre (-0.1732, -0.0016) ccw
  line L185 (-22.7347, 5.2911) -> (-21.7892, 5.1124)
  line L186 (-22.3583, 6.6956) -> (-21.4502, 6.3776)
  arc A235 (-23.9994, 6.1296) -> (-22.7347, 5.2911) centre (-22.7878, 6.5841) ccw
  arc A236 (-23.8729, 6.6019) -> (-23.9994, 6.1296) centre (-0.1732, -0.0016) ccw
  arc A237 (-22.3583, 6.6956) -> (-23.8729, 6.6019) centre (-23.0509, 5.6024) ccw
  line L187 (-21.3636, 6.7154) -> (-21.3426, 6.7069)
  line L188 (-22.3092, 1.7718) -> (-22.301, 1.7707) construction
  arc A238 (-22.1229, 3.4068) -> (-22.2571, 2.3872) centre (-0.1732, -0.0016) ccw
  arc A239 (-22.1009, 3.5458) -> (-22.2718, 2.2472) centre (-0.1732, -0.0016) ccw
  line L189 (-23.2325, 2.301) -> (-22.2718, 2.2472)
  line L190 (-23.0427, 3.7426) -> (-22.1009, 3.5458)
  arc A240 (-24.5959, 2.9672) -> (-23.2325, 2.301) centre (-23.454, 3.576) ccw
  arc A241 (-24.5321, 3.4519) -> (-24.5959, 2.9672) centre (-0.1732, -0.0016) ccw
  arc A242 (-23.0427, 3.7426) -> (-24.5321, 3.4519) centre (-23.5866, 2.5683) ccw
  line L191 (-22.059, 3.892) -> (-22.0371, 3.8863)
  dimension "d42" = 360
  constraints: 482 point on circle, 384 end point, 242 centre point, 3 coincident, 1 concentric, 1 horizontal, 1249 other
extrude "Extrusion7" add sketch "Sketch4" along normal blind 7
sketch "Sketch5" plane through (25.4, 0, 0) normal (1, 0, 0) x (0, 0, -1)
  circle A0 centre (0, 0) radius 4.445 projected
  circle A1 centre (0, 0) radius 11.176
  dimension "d48" = 22.352
  constraints: 1 centre point, 1 coincident
  measures "d48" diameter of A1
extrude "Extrusion8" cut sketch "Sketch5" against normal up to surface (6.858 mm away)
sketch "Sketch6" plane through (-7, 9.1003, 20.0892) normal (0, 0.8926, -0.4508) x (1, 0, 0)
  point P0 (7, 22.0345)
sketch "Sketch7" plane through (-7, 0, 0) normal (-1, 0, 0) x (0, 0, 1)
  circle A0 centre (0, 0) radius 11.176
  dimension "d51" = 22.352
  constraints: 1 centre point, 1 coincident
  measures "d51" diameter of A0
extrude "Extrusion9" cut sketch "Sketch7" against normal up to surface (13.858 mm away)
body "Solid1"
